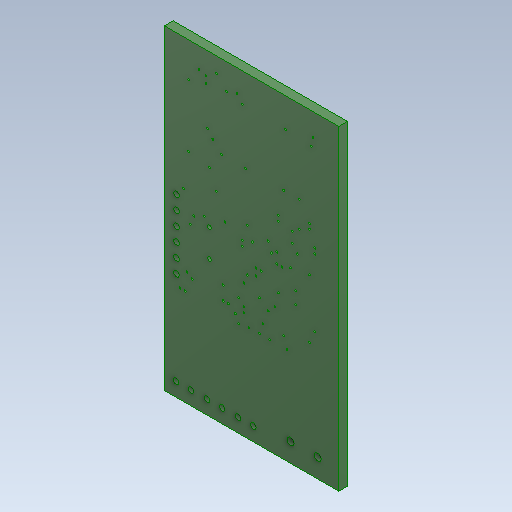
# Autodesk Inventor part: Dog_driver.brd_Outline
Saved by Autodesk Inventor 2020 (Build 240168000, 168)
## iProperties
Created: 2019-05-24
Part Number: Dog_driver.brd_Outline
Material: Generic
Document SubType Name: Modeling
Designer: psrob
Density: 1 g/cm^3
Appearance: Board Outline
Author: psrob
Autodesk Inventor part; units mm, degrees
ref_plane "YZ Plane" through (0, 0, 0) normal (1, 0, 0) x (0, 1, 0)
ref_plane "XZ Plane" through (0, 0, 0) normal (0, 1, 0) x (-1, 0, 0)
ref_plane "XY Plane" through (0, 0, 0) normal (0, 0, 1) x (1, 0, 0)
sketch "Sketch1" plane through (0, 0, 0) normal (0, 0, 1) x (1, 0, 0)
  line L0 (0, 0) -> (32.0475, 0)
  line L1 (32.0475, 0) -> (32.0475, 58.09)
  line L2 (32.0475, 58.09) -> (0, 58.09)
  line L3 (0, 58.09) -> (0, 0)
  circle A0 centre (2.22, 19.69) radius 0.51
  circle A1 centre (2.22, 22.23) radius 0.51
  circle A2 centre (2.22, 24.77) radius 0.51
  circle A3 centre (2.22, 27.3) radius 0.51
  circle A4 centre (2.22, 29.85) radius 0.51
  circle A5 centre (2.22, 32.38) radius 0.51
  circle A6 centre (7.81, 2.54) radius 0.51
  circle A7 centre (10.6, 2.54) radius 0.51
  circle A8 centre (16.32, 2.54) radius 0.51
  circle A9 centre (13.53, 2.54) radius 0.51
  circle A10 centre (2.1, 2.54) radius 0.51
  circle A11 centre (4.89, 2.54) radius 0.51
  circle A12 centre (23.18, 3.49) radius 0.65
  circle A13 centre (28.18, 3.49) radius 0.65
  circle A14 centre (8.26, 25.08) radius 0.35
  circle A15 centre (8.26, 30.16) radius 0.35
  circle A16 centre (23.495, 35.2425) radius 0.175
  circle A17 centre (24.4475, 33.9725) radius 0.175
  circle A18 centre (24.765, 38.1) radius 0.175
  circle A19 centre (26.67, 39.0525) radius 0.175
  circle A20 centre (20.955, 37.465) radius 0.175
  circle A21 centre (8.255, 39.6875) radius 0.175
  circle A22 centre (23.495, 37.1475) radius 0.175
  circle A23 centre (4.445, 40.3225) radius 0.175
  circle A24 centre (20.6375, 32.385) radius 0.175
  circle A25 centre (26.67, 20.955) radius 0.175
  circle A26 centre (20.955, 38.4175) radius 0.175
  circle A27 centre (27.6225, 36.5125) radius 0.175
  circle A28 centre (14.2875, 31.115) radius 0.175
  circle A29 centre (20.6375, 30.48) radius 0.175
  circle A30 centre (14.2875, 52.705) radius 0.175
  circle A31 centre (4.445, 51.7525) radius 0.175
  circle A32 centre (16.8275, 27.94) radius 0.175
  circle A33 centre (14.2875, 30.1625) radius 0.175
  circle A34 centre (13.335, 53.975) radius 0.175
  circle A35 centre (7.62, 53.975) radius 0.175
  circle A36 centre (15.24, 33.9725) radius 0.175
  circle A37 centre (7.62, 52.705) radius 0.175
  circle A38 centre (22.225, 52.705) radius 0.175
  circle A39 centre (7.9375, 45.72) radius 0.175
  circle A40 centre (4.7625, 28.8925) radius 0.175
  circle A41 centre (20.955, 26.035) radius 0.175
  circle A42 centre (26.9875, 52.3875) radius 0.175
  circle A43 centre (3.4925, 33.9725) radius 0.175
  circle A44 centre (19.3675, 17.78) radius 0.175
  circle A45 centre (13.0175, 18.7325) radius 0.175
  circle A46 centre (27.6225, 35.56) radius 0.175
  circle A47 centre (19.05, 33.3375) radius 0.175
  circle A48 centre (24.765, 42.8625) radius 0.175
  circle A49 centre (11.1125, 32.385) radius 0.175
  circle A50 centre (27.6225, 23.1775) radius 0.175
  circle A51 centre (17.4625, 23.495) radius 0.175
  circle A52 centre (16.8275, 26.67) radius 0.175
  circle A53 centre (10.795, 19.685) radius 0.175
  circle A54 centre (15.5575, 17.78) radius 0.175
  circle A55 centre (18.0975, 19.685) radius 0.175
  circle A56 centre (21.9075, 19.685) radius 0.175
  circle A57 centre (19.05, 22.225) radius 0.175
  circle A58 centre (4.1275, 20.955) radius 0.175
  circle A59 centre (9.525, 55.245) radius 0.175
  circle A60 centre (26.67, 31.75) radius 0.175
  circle A61 centre (10.795, 22.225) radius 0.175
  circle A62 centre (13.6525, 21.59) radius 0.175
  circle A63 centre (13.6525, 17.4625) radius 0.175
  circle A64 centre (17.4625, 17.78) radius 0.175
  circle A65 centre (11.7475, 19.685) radius 0.175
  circle A66 centre (14.605, 19.685) radius 0.175
  circle A67 centre (20.32, 23.495) radius 0.175
  circle A68 centre (3.81, 17.78) radius 0.175
  circle A69 centre (22.5425, 17.78) radius 0.175
  circle A70 centre (2.8575, 17.78) radius 0.175
  circle A71 centre (23.1775, 31.115) radius 0.175
  circle A72 centre (17.78, 27.94) radius 0.175
  circle A73 centre (27.305, 53.975) radius 0.175
  circle A74 centre (11.43, 53.34) radius 0.175
  circle A75 centre (6.35, 54.2925) radius 0.175
  circle A76 centre (15.24, 26.035) radius 0.175
  circle A77 centre (24.13, 27.94) radius 0.175
  circle A78 centre (24.13, 25.7175) radius 0.175
  circle A79 centre (14.605, 24.4475) radius 0.175
  circle A80 centre (26.67, 40.005) radius 0.175
  circle A81 centre (21.9075, 42.8625) radius 0.175
  circle A82 centre (8.89, 44.45) radius 0.175
  circle A83 centre (14.605, 20.6375) radius 0.175
  circle A84 centre (5.08, 20.32) radius 0.175
  circle A85 centre (16.1925, 31.75) radius 0.175
  circle A86 centre (7.3025, 31.4325) radius 0.175
  circle A87 centre (21.59, 30.48) radius 0.175
  circle A88 centre (5.3975, 30.48) radius 0.175
  circle A89 centre (19.685, 31.75) radius 0.175
  circle A90 centre (10.4775, 42.8625) radius 0.175
  circle A91 centre (14.9225, 42.8625) radius 0.175
  circle A92 centre (9.525, 36.5125) radius 0.175
  constraints: 93 centre point, 8 end point
extrude "Dog_driver.brd_Outline" add sketch "Sketch1" along normal blind 1.6
body "Solid1"
